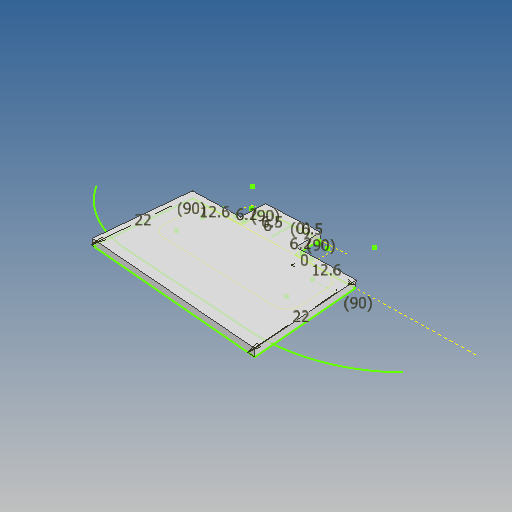
# Autodesk Inventor part: ELE-PRT-3001-Dummy_Power_Monitor
Saved by Autodesk Inventor 2026 (Build 300175000, 175)
## iProperties
Created: 2026-07-24
Part Number: ELE-PRT-3001-Dummy_Power_Monitor
Material: Generic
Document SubType Name: Modeling
Designer: Pacman Ng
Density: 1 g/cm^3
Appearance: Default
Author: Pacman Ng
Autodesk Inventor part; units mm, degrees
ref_plane "YZ Plane" through (0, 0, 0) normal (1, 0, 0) x (0, 1, 0)
ref_plane "XZ Plane" through (0, 0, 0) normal (0, 1, 0) x (-1, 0, 0)
ref_plane "XY Plane" through (0, 0, 0) normal (0, 0, 1) x (1, 0, 0)
sketch "Sketch2" plane through (0, 0, 0) normal (0, 0, 1) x (1, 0, 0)
  arc A0 (-42.2846, -11.2117) -> (-21.43, -19.85) centre (-21.43, 9.6429) ccw
  line L0 (7.43, -19.85) -> (-21.43, -19.85)
  arc A1 (7.43, -19.85) -> (28.2846, -11.2117) centre (7.43, 9.6429) ccw
  line L1 (9, -10.25) -> (9, -4.25) construction
  arc A2 (6, -13.25) -> (9, -10.25) centre (6, -10.25) ccw construction
  line L2 (-20, -13.25) -> (6, -13.25) construction
  arc A3 (-23, -10.25) -> (-20, -13.25) centre (-20, -10.25) ccw construction
  line L3 (-23, -4.25) -> (-23, -10.25) construction
  arc A4 (-20, -1.25) -> (-23, -4.25) centre (-20, -4.25) ccw construction
  line L4 (6, -1.25) -> (-20, -1.25) construction
  arc A5 (9, -4.25) -> (6, -1.25) centre (6, -4.25) ccw construction
  line L5 (-16, -1) -> (-14, -1) construction
  arc A6 (-17, 0) -> (-16, -1) centre (-16, 0) ccw construction
  line L6 (-17, 4) -> (-17, 0) construction
  arc A7 (-16, 5) -> (-17, 4) centre (-16, 4) ccw construction
  line L7 (-14, 5) -> (-16, 5) construction
  arc A8 (-13, 4) -> (-14, 5) centre (-14, 4) ccw construction
  line L8 (-13, 0) -> (-13, 4) construction
  arc A9 (-14, -1) -> (-13, 0) centre (-14, 0) ccw construction
  line L9 (0, -1) -> (2, -1) construction
  arc A10 (-1, 0) -> (0, -1) centre (0, 0) ccw construction
  line L10 (-1, 4) -> (-1, 0) construction
  arc A11 (0, 5) -> (-1, 4) centre (0, 4) ccw construction
  line L11 (2, 5) -> (0, 5) construction
  arc A12 (3, 4) -> (2, 5) centre (2, 4) ccw construction
  line L12 (3, 0) -> (3, 4) construction
  arc A13 (2, -1) -> (3, 0) centre (2, 0) ccw construction
  line L13 (-7, 0) -> (-7, 5)
  line L14 (-7, 5) -> (-0.5, 5)
  line L15 (-7, 5) -> (-0.5, 5) construction
  line L16 (-7, 5) -> (-13.5, 5)
  line L17 (-13.5, 5) -> (-13.5, -1.2)
  line L18 (-13.5, 5) -> (-7.3, 5) construction
  line L19 (-0.5, 5) -> (-0.5, -1.2)
  line L20 (-0.5, 5) -> (5.7, 5) construction
  line L21 (-13.5, -1.2) -> (-26.1, -1.2)
  line L22 (-0.5, -1.2) -> (12.1, -1.2)
  line L23 (-0.5, -1.2) -> (12.1, -1.2) construction
  line L24 (-26.1, -1.2) -> (-26.1, -23.2)
  line L25 (-26.1, -1.2) -> (-4.1, -1.2) construction
  line L26 (12.1, -1.2) -> (12.1, -23.2)
  line L27 (12.1, -1.2) -> (34.1, -1.2) construction
  line L28 (12.1, -23.2) -> (-26.1, -23.2)
  point P0 (0, 0)
  dimension "d0" = 6
  dimension "d1" = 6.5
  dimension "d2" = 0
  dimension "d3" = 6.5
  dimension "d4" = 6.2
  dimension "d5" = 90
  dimension "d6" = 6.2
  dimension "d7" = 90
  dimension "d8" = 12.6
  dimension "d9" = 12.6
  dimension "d10" = 0
  dimension "d11" = 22
  dimension "d12" = 90
  dimension "d13" = 22
  dimension "d14" = 90
  constraints: 58 end point, 28 point on circle, 14 centre point, 8 horizontal, 6 equal length, 3 parallel, 3 vertical, 1 perpendicular
  measures "d0" distance between parallel lines of L8 L13
  measures "d1" distance of L13.end L14.end
  measures "d2" distance between parallel lines of L14 L15
  measures "d3" distance of L13.end L16.end
  measures "d4" distance of L16.end L17.end
  measures "d5" angle of L17 L18
  measures "d6" distance of L15.end L19.end
  measures "d7" angle of L19 L20
  measures "d8" distance of L17.end L21.end
  measures "d9" distance of L19.end L22.end
  measures "d10" distance between parallel lines of L23 L22
  measures "d11" distance of L21.end L24.end
  measures "d12" angle of L24 L25
  measures "d13" distance of L23.end L26.end
  measures "d14" angle of L26 L27
extrude "Extrusion1" add sketch "Sketch2" along normal blind 1.6
body "Solid1"
